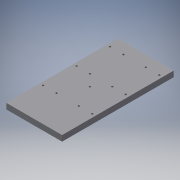
# Autodesk Inventor part: BLOCO_SUPORTE_SPINDLE
Saved by Autodesk Inventor 2018 (Build 220112000, 112)
## iProperties
Created: 2018-10-10
Part Number: BLOCO_SUPORTE_SPINDLE
Material: Genérico
Document SubType Name: Modeling
Designer: Usuário
Density: 1 g/cm^3
Appearance: Padrão
Mass: 396.875 g
Surface Area: 720.25 cm^2
Volume: 396.875 cm^3
Author: Usuário
Autodesk Inventor part; units mm, degrees
ref_plane "YZ Plane" through (0, 0, 0) normal (1, 0, 0) x (0, 1, 0)
ref_plane "XZ Plane" through (0, 0, 0) normal (0, 1, 0) x (-1, 0, 0)
ref_plane "XY Plane" through (0, 0, 0) normal (0, 0, 1) x (1, 0, 0)
sketch "Esboço1" plane through (0, 0, 0) normal (0, 0, 1) x (1, 0, 0)
  line L0 (-62.5, 125) -> (62.5, 125)
  line L1 (62.5, 125) -> (62.5, -125)
  line L2 (62.5, -125) -> (-62.5, -125)
  line L3 (-62.5, -125) -> (-62.5, 125)
  line L4 (-62.5, 125) -> (62.5, -125) construction
  line L5 (62.5, 125) -> (-62.5, -125) construction
  point P0 (0, 0)
  dimension "d0" = 125
  dimension "d1" = 250
  constraints: 12 end point, 2 midpoint, 2 parallel, 1 horizontal, 1 perpendicular
  measures "d0" distance of L1.end L2.end
  measures "d1" distance of L0.end L1.end
extrude "Extrusão1" add sketch "Esboço1" along normal blind 12.7
sketch "Esboço4" plane through (0, 0, 0) normal (0, 0, -1) x (-1, 0, 0)
  circle A0 centre (-25, 100) radius 2.75 construction
  circle A1 centre (-55, 100) radius 2.75 construction
  circle A2 centre (25, 100) radius 2.75 construction
  circle A3 centre (55, 100) radius 2.75 construction
  circle A4 centre (55, 25) radius 2.75 construction
  circle A5 centre (25, 25) radius 2.75 construction
  circle A6 centre (55, -50) radius 2.75 construction
  circle A7 centre (25, -50) radius 2.75 construction
  circle A8 centre (-25, -50) radius 2.75 construction
  circle A9 centre (-55, -50) radius 2.75 construction
  circle A10 centre (-25, 25) radius 2.75 construction
  circle A11 centre (-55, 25) radius 2.75 construction
  point P0 (0, 0)
  constraints: 12 centre point
hole "Furo1" at (0, 0, 0) at (25, 100, 0) at (55, 100, 0) at (-25, 100, 0) at (-55, 100, 0) at (-55, 25, 0) at (-25, 25, 0) at (-55, -50, 0) at (-25, -50, 0) at (25, -50, 0) at (55, -50, 0) at (25, 25, 0) at (55, 25, 0) direction (0, 0, 1) diameter 4.134 end through all thread size "M5x0.8" class "6H" standard "ISO Metric profile"
sketch "Esboço5" plane through (-62.5, 125, 0) normal (0, 1, 0) x (1, 0, 0)
  line L0 (0, 0) -> (0, -12.7) construction
  line L1 (0, -6.35) -> (125, -6.35) construction
  line L2 (125, 0) -> (125, -12.7) construction
  circle A0 centre (62.5, -6.35) radius 2 construction
  circle A1 centre (90.5, -6.35) radius 2 construction
  circle A2 centre (118.5, -6.35) radius 2 construction
  circle A3 centre (34.5, -6.35) radius 2 construction
  circle A4 centre (62.5, -6.35) radius 2 construction
  circle A5 centre (90.5, -6.35) radius 2 construction
  circle A6 centre (6.5, -6.35) radius 2 construction
  circle A7 centre (34.5, -6.35) radius 2 construction
  circle A8 centre (62.5, -6.35) radius 2 construction
  point P0 (62.5, 0)
  dimension "d11" = 4
  dimension "d14" = 28
  dimension "d17" = 28
  dimension "d28" = 62.5
  constraints: 9 centre point, 2 end point, 2 horizontal, 2 midpoint, 16 other
  measures "d11" diameter of A0
  measures "d14" distance of A0.centre A1.centre
  measures "d17" distance of A0.centre A3.centre
  measures "d28" distance from line of L0 A0.centre
hole "Furo2" at (-56, 125, 6.35) at (-28, 125, 6.35) at (0, 125, 6.35) at (28, 125, 6.35) at (56, 125, 6.35) direction (0, -1, 0) diameter 4.134 depth 15 tip angle 118 thread size "M5x0.8" class "6H" standard "ISO Metric profile"
